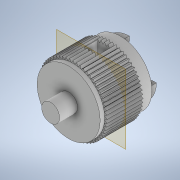
# Autodesk Inventor part: PotAttachmentB10L
Saved by Autodesk Inventor 2022 (Build 260153000, 153)
## iProperties
Created: 2021-10-23
Part Number: PotAttachmentB10L
Material: Generic
Document SubType Name: Modeling
Designer: teh18
Density: 1 g/cm^3
Appearance: Default
Author: teh18
Autodesk Inventor part; units mm, degrees
ref_plane "YZ Plane" through (0, 0, 0) normal (1, 0, 0) x (0, 1, 0)
ref_plane "XZ Plane" through (0, 0, 0) normal (0, 1, 0) x (-1, 0, 0)
ref_plane "XY Plane" through (0, 0, 0) normal (0, 0, 1) x (1, 0, 0)
sketch "Sketch1" plane through (0, 0, 0) normal (0, 0, 1) x (1, 0, 0)
  arc A0 (-0.1225, 6.9989) -> (-6, 3.6056) centre (0, 0) ccw projected
  circle A1 centre (0, 0) radius 7
  line L0 (0, -12) -> (0, -10) projected
  arc A2 (0, -10) -> (10, 0) centre (0, 0) ccw projected
  line L1 (10, 0) -> (12, 0) projected
  arc A3 (0, -12) -> (12, 0) centre (0, 0) ccw projected
  line L2 (0, 12) -> (0, 10) projected
  arc A4 (0, 10) -> (-10, 0) centre (0, 0) ccw projected
  line L3 (-10, 0) -> (-12, 0) projected
  arc A5 (0, 12) -> (-12, 0) centre (0, 0) ccw projected
  arc A6 (4.4269, -19.95) -> (6.1412, -19.4907) centre (5.1647, -19.275) ccw projected
  arc A7 (13.8088, -15.0638) -> (6.1412, -19.4907) centre (12, -20.7846) ccw projected
  arc A8 (13.8088, -15.0638) -> (15.0638, -13.8088) centre (14.1103, -14.1103) ccw projected
  arc A9 (19.4907, -6.1412) -> (15.0638, -13.8088) centre (20.7846, -12) ccw projected
  arc A10 (19.4907, -6.1412) -> (19.95, -4.4269) centre (19.275, -5.1647) ccw projected
  arc A11 (27.8571, 4.5959) -> (19.95, -4.4269) centre (24, 0) ccw projected
  arc A12 (27.8571, 4.5959) -> (29.4828, 5.5468) centre (28.5, 5.3619) ccw projected
  arc A13 (29.4828, 5.5468) -> (27.5804, 11.8035) centre (0, 0) ccw projected
  line L4 (27.5804, 11.8035) -> (33.0964, 14.1643) projected
  arc A14 (33.0964, 14.1643) -> (26.445, 24.4267) centre (0, 0) ccw projected
  line L5 (26.445, 24.4267) -> (22.0375, 20.3556) projected
  arc A15 (22.0375, 20.3556) -> (-20.3556, 22.0375) centre (0, 0) ccw projected
  line L6 (-20.3556, 22.0375) -> (-16.2845, 17.63) projected
  arc A16 (-16.2845, 17.63) -> (-5.9529, -23.25) centre (0, 0) ccw projected
  arc A17 (4.4269, -19.95) -> (-5.9529, -23.25) centre (0, -24) ccw projected
  arc A18 (-1, 6.9282) -> (-6.9282, 1) centre (0, 0) ccw projected
  line L7 (-1, 6.9282) -> (-1, 1) projected
  line L8 (-1, 1) -> (-6.9282, 1) projected
  line L9 (-6.9282, -1) -> (-1, -1) projected
  line L10 (-1, -1) -> (-1, -6.9282) projected
  arc A19 (-6.9282, -1) -> (-1, -6.9282) centre (0, 0) ccw projected
  line L11 (1, -6.9282) -> (1, -1) projected
  line L12 (1, -1) -> (6.9282, -1) projected
  arc A20 (1, -6.9282) -> (6.9282, -1) centre (0, 0) ccw projected
  line L13 (6.9282, 1) -> (1, 1) projected
  line L14 (1, 1) -> (1, 6.9282) projected
  arc A21 (6.9282, 1) -> (1, 6.9282) centre (0, 0) ccw projected
  circle A22 centre (0, 0) radius 14
  point P0 (0, 0)
  point P1 (-6, 3.6056)
  point P2 (-0.1225, 6.9989)
  dimension "d2" = 28
  constraints: 1 centre point, 1 coincident, 2 other
  measures "d2" diameter of A22
extrude "Extrusion1" add sketch "Sketch1" along normal blind 23 contours L0 A2 L1 A3 | L2 A4 L3 A5 | A22
sketch "Sketch2" plane through (0, 0, 0) normal (0, 0, -1) x (-1, 0, 0)
  line L0 (0, -12) -> (0, -10) projected
  arc A0 (-10, 0) -> (0, -10) centre (0, 0) ccw projected
  line L1 (-10, 0) -> (-12, 0) projected
  arc A1 (-12, 0) -> (0, -12) centre (0, 0) ccw projected
  line L2 (0, 12) -> (0, 10) projected
  arc A2 (10, 0) -> (0, 10) centre (0, 0) ccw projected
  line L3 (10, 0) -> (12, 0) projected
  arc A3 (12, 0) -> (0, 12) centre (0, 0) ccw projected
  arc A4 (-6.1412, -19.4907) -> (-4.4269, -19.95) centre (-5.1647, -19.275) ccw projected
  arc A5 (-6.1412, -19.4907) -> (-13.8088, -15.0638) centre (-12, -20.7846) ccw projected
  arc A6 (-15.0638, -13.8088) -> (-13.8088, -15.0638) centre (-14.1103, -14.1103) ccw projected
  arc A7 (-15.0638, -13.8088) -> (-19.4907, -6.1412) centre (-20.7846, -12) ccw projected
  arc A8 (-19.95, -4.4269) -> (-19.4907, -6.1412) centre (-19.275, -5.1647) ccw projected
  arc A9 (-19.95, -4.4269) -> (-27.8571, 4.5959) centre (-24, 0) ccw projected
  arc A10 (-29.4828, 5.5468) -> (-27.8571, 4.5959) centre (-28.5, 5.3619) ccw projected
  arc A11 (-27.5804, 11.8035) -> (-29.4828, 5.5468) centre (0, 0) ccw projected
  line L4 (-27.5804, 11.8035) -> (-33.0964, 14.1643) projected
  arc A12 (-26.445, 24.4267) -> (-33.0964, 14.1643) centre (0, 0) ccw projected
  line L5 (-26.445, 24.4267) -> (-22.0375, 20.3556) projected
  arc A13 (20.3556, 22.0375) -> (-22.0375, 20.3556) centre (0, 0) ccw projected
  line L6 (20.3556, 22.0375) -> (16.2845, 17.63) projected
  arc A14 (5.9529, -23.25) -> (16.2845, 17.63) centre (0, 0) ccw projected
  arc A15 (5.9529, -23.25) -> (-4.4269, -19.95) centre (0, -24) ccw projected
  arc A16 (6.9282, 1) -> (1, 6.9282) centre (0, 0) ccw projected
  line L7 (1, 6.9282) -> (1, 1) projected
  line L8 (1, 1) -> (6.9282, 1) projected
  line L9 (6.9282, -1) -> (1, -1) projected
  line L10 (1, -1) -> (1, -6.9282) projected
  arc A17 (1, -6.9282) -> (6.9282, -1) centre (0, 0) ccw projected
  line L11 (-1, -6.9282) -> (-1, -1) projected
  line L12 (-1, -1) -> (-6.9282, -1) projected
  arc A18 (-6.9282, -1) -> (-1, -6.9282) centre (0, 0) ccw projected
  line L13 (-6.9282, 1) -> (-1, 1) projected
  line L14 (-1, 1) -> (-1, 6.9282) projected
  arc A19 (-1, 6.9282) -> (-6.9282, 1) centre (0, 0) ccw projected
  point P0 (0, 0)
extrude "Extrusion2" add sketch "Sketch2" along normal blind 4 contours A1 L1 A0 L0 | A3 L3 A2 L2
ref_plane "Work Plane1" through (0, 0, 13) normal (0, 0, 1) x (1, 0, 0)
sketch "Sketch4" plane through (0, 0, 13) normal (0, 0, 1) x (1, 0, 0)
  circle A0 centre (0, 0) radius 3
  circle A1 centre (0, 0) radius 7 projected
  dimension "d10" = 6
  constraints: 1 centre point, 1 coincident
  measures "d10" diameter of A0
extrude "Extrusion4" add sketch "Sketch4" along normal up to surface (10 mm away) contours A0 | A1
sketch "Sketch6" plane through (0, 0, 23) normal (0, 0, 1) x (1, 0, 0)
  circle A0 centre (0, 0) radius 4
  dimension "d25" = 8
  constraints: 1 centre point, 1 coincident
  measures "d25" diameter of A0
extrude "Extrusion6" add sketch "Sketch6" along normal blind 8
sketch "Sketch7" plane through (0, 0, 13) normal (0, 0, 1) x (1, 0, 0)
  circle A0 centre (0, 0) radius 14 projected
  line L0 (0, 15.1547) -> (1, 13.4226)
  line L1 (1, 13.4226) -> (-1, 13.4226)
  line L2 (-1, 13.4226) -> (0, 15.1547)
  line L3 (-1.5841, 15.0717) -> (-0.4085, 13.4536)
  line L4 (-2.3976, 13.2446) -> (-1.5841, 15.0717)
  line L5 (-0.4085, 13.4536) -> (-2.3976, 13.2446)
  line L6 (-3.1508, 14.8235) -> (-1.8126, 13.3372)
  line L7 (-3.7689, 12.9214) -> (-3.1508, 14.8235)
  line L8 (-1.8126, 13.3372) -> (-3.7689, 12.9214)
  line L9 (-4.6831, 14.413) -> (-3.1968, 13.0747)
  line L10 (-5.0989, 12.4567) -> (-4.6831, 14.413)
  line L11 (-3.1968, 13.0747) -> (-5.0989, 12.4567)
  line L12 (-6.164, 13.8445) -> (-4.5459, 12.6689)
  line L13 (-6.373, 11.8555) -> (-6.164, 13.8445)
  line L14 (-4.5459, 12.6689) -> (-6.373, 11.8555)
  line L15 (-7.5774, 13.1244) -> (-5.8453, 12.1244)
  line L16 (-7.5774, 11.1244) -> (-7.5774, 13.1244)
  line L17 (-5.8453, 12.1244) -> (-7.5774, 11.1244)
  line L18 (-8.9077, 12.2604) -> (-7.0806, 11.4469)
  line L19 (-8.6987, 10.2714) -> (-8.9077, 12.2604)
  line L20 (-7.0806, 11.4469) -> (-8.6987, 10.2714)
  line L21 (-10.1405, 11.2621) -> (-8.2384, 10.6441)
  line L22 (-9.7247, 9.3058) -> (-10.1405, 11.2621)
  line L23 (-8.2384, 10.6441) -> (-9.7247, 9.3058)
  line L24 (-11.2621, 10.1405) -> (-9.3058, 9.7247)
  line L25 (-10.6441, 8.2384) -> (-11.2621, 10.1405)
  line L26 (-9.3058, 9.7247) -> (-10.6441, 8.2384)
  line L27 (-12.2604, 8.9077) -> (-10.2714, 8.6987)
  line L28 (-11.4469, 7.0806) -> (-12.2604, 8.9077)
  line L29 (-10.2714, 8.6987) -> (-11.4469, 7.0806)
  line L30 (-13.1244, 7.5774) -> (-11.1244, 7.5774)
  line L31 (-12.1244, 5.8453) -> (-13.1244, 7.5774)
  line L32 (-11.1244, 7.5774) -> (-12.1244, 5.8453)
  line L33 (-13.8445, 6.164) -> (-11.8555, 6.373)
  line L34 (-12.6689, 4.5459) -> (-13.8445, 6.164)
  line L35 (-11.8555, 6.373) -> (-12.6689, 4.5459)
  line L36 (-14.413, 4.6831) -> (-12.4567, 5.0989)
  line L37 (-13.0747, 3.1968) -> (-14.413, 4.6831)
  line L38 (-12.4567, 5.0989) -> (-13.0747, 3.1968)
  line L39 (-14.8235, 3.1508) -> (-12.9214, 3.7689)
  line L40 (-13.3372, 1.8126) -> (-14.8235, 3.1508)
  line L41 (-12.9214, 3.7689) -> (-13.3372, 1.8126)
  line L42 (-15.0717, 1.5841) -> (-13.2446, 2.3976)
  line L43 (-13.4536, 0.4085) -> (-15.0717, 1.5841)
  line L44 (-13.2446, 2.3976) -> (-13.4536, 0.4085)
  line L45 (-15.1547, 0) -> (-13.4226, 1)
  line L46 (-13.4226, -1) -> (-15.1547, 0)
  line L47 (-13.4226, 1) -> (-13.4226, -1)
  line L48 (-15.0717, -1.5841) -> (-13.4536, -0.4085)
  line L49 (-13.2446, -2.3976) -> (-15.0717, -1.5841)
  line L50 (-13.4536, -0.4085) -> (-13.2446, -2.3976)
  line L51 (-14.8235, -3.1508) -> (-13.3372, -1.8126)
  line L52 (-12.9214, -3.7689) -> (-14.8235, -3.1508)
  line L53 (-13.3372, -1.8126) -> (-12.9214, -3.7689)
  line L54 (-14.413, -4.6831) -> (-13.0747, -3.1968)
  line L55 (-12.4567, -5.0989) -> (-14.413, -4.6831)
  line L56 (-13.0747, -3.1968) -> (-12.4567, -5.0989)
  line L57 (-13.8445, -6.164) -> (-12.6689, -4.5459)
  line L58 (-11.8555, -6.373) -> (-13.8445, -6.164)
  line L59 (-12.6689, -4.5459) -> (-11.8555, -6.373)
  line L60 (-13.1244, -7.5774) -> (-12.1244, -5.8453)
  line L61 (-11.1244, -7.5774) -> (-13.1244, -7.5774)
  line L62 (-12.1244, -5.8453) -> (-11.1244, -7.5774)
  line L63 (-12.2604, -8.9077) -> (-11.4469, -7.0806)
  line L64 (-10.2714, -8.6987) -> (-12.2604, -8.9077)
  line L65 (-11.4469, -7.0806) -> (-10.2714, -8.6987)
  line L66 (-11.2621, -10.1405) -> (-10.6441, -8.2384)
  line L67 (-9.3058, -9.7247) -> (-11.2621, -10.1405)
  line L68 (-10.6441, -8.2384) -> (-9.3058, -9.7247)
  line L69 (-10.1405, -11.2621) -> (-9.7247, -9.3058)
  line L70 (-8.2384, -10.6441) -> (-10.1405, -11.2621)
  line L71 (-9.7247, -9.3058) -> (-8.2384, -10.6441)
  line L72 (-8.9077, -12.2604) -> (-8.6987, -10.2714)
  line L73 (-7.0806, -11.4469) -> (-8.9077, -12.2604)
  line L74 (-8.6987, -10.2714) -> (-7.0806, -11.4469)
  line L75 (-7.5774, -13.1244) -> (-7.5774, -11.1244)
  line L76 (-5.8453, -12.1244) -> (-7.5774, -13.1244)
  line L77 (-7.5774, -11.1244) -> (-5.8453, -12.1244)
  line L78 (-6.164, -13.8445) -> (-6.373, -11.8555)
  line L79 (-4.5459, -12.6689) -> (-6.164, -13.8445)
  line L80 (-6.373, -11.8555) -> (-4.5459, -12.6689)
  line L81 (-4.6831, -14.413) -> (-5.0989, -12.4567)
  line L82 (-3.1968, -13.0747) -> (-4.6831, -14.413)
  line L83 (-5.0989, -12.4567) -> (-3.1968, -13.0747)
  line L84 (-3.1508, -14.8235) -> (-3.7689, -12.9214)
  line L85 (-1.8126, -13.3372) -> (-3.1508, -14.8235)
  line L86 (-3.7689, -12.9214) -> (-1.8126, -13.3372)
  line L87 (-1.5841, -15.0717) -> (-2.3976, -13.2446)
  line L88 (-0.4085, -13.4536) -> (-1.5841, -15.0717)
  line L89 (-2.3976, -13.2446) -> (-0.4085, -13.4536)
  line L90 (0, -15.1547) -> (-1, -13.4226)
  line L91 (1, -13.4226) -> (0, -15.1547)
  line L92 (-1, -13.4226) -> (1, -13.4226)
  line L93 (1.5841, -15.0717) -> (0.4085, -13.4536)
  line L94 (2.3976, -13.2446) -> (1.5841, -15.0717)
  line L95 (0.4085, -13.4536) -> (2.3976, -13.2446)
  line L96 (3.1508, -14.8235) -> (1.8126, -13.3372)
  line L97 (3.7689, -12.9214) -> (3.1508, -14.8235)
  line L98 (1.8126, -13.3372) -> (3.7689, -12.9214)
  line L99 (4.6831, -14.413) -> (3.1968, -13.0747)
  line L100 (5.0989, -12.4567) -> (4.6831, -14.413)
  line L101 (3.1968, -13.0747) -> (5.0989, -12.4567)
  line L102 (6.164, -13.8445) -> (4.5459, -12.6689)
  line L103 (6.373, -11.8555) -> (6.164, -13.8445)
  line L104 (4.5459, -12.6689) -> (6.373, -11.8555)
  line L105 (7.5774, -13.1244) -> (5.8453, -12.1244)
  line L106 (7.5774, -11.1244) -> (7.5774, -13.1244)
  line L107 (5.8453, -12.1244) -> (7.5774, -11.1244)
  line L108 (8.9077, -12.2604) -> (7.0806, -11.4469)
  line L109 (8.6987, -10.2714) -> (8.9077, -12.2604)
  line L110 (7.0806, -11.4469) -> (8.6987, -10.2714)
  line L111 (10.1405, -11.2621) -> (8.2384, -10.6441)
  line L112 (9.7247, -9.3058) -> (10.1405, -11.2621)
  line L113 (8.2384, -10.6441) -> (9.7247, -9.3058)
  line L114 (11.2621, -10.1405) -> (9.3058, -9.7247)
  line L115 (10.6441, -8.2384) -> (11.2621, -10.1405)
  line L116 (9.3058, -9.7247) -> (10.6441, -8.2384)
  line L117 (12.2604, -8.9077) -> (10.2714, -8.6987)
  line L118 (11.4469, -7.0806) -> (12.2604, -8.9077)
  line L119 (10.2714, -8.6987) -> (11.4469, -7.0806)
  line L120 (13.1244, -7.5774) -> (11.1244, -7.5774)
  line L121 (12.1244, -5.8453) -> (13.1244, -7.5774)
  line L122 (11.1244, -7.5774) -> (12.1244, -5.8453)
  line L123 (13.8445, -6.164) -> (11.8555, -6.373)
  line L124 (12.6689, -4.5459) -> (13.8445, -6.164)
  line L125 (11.8555, -6.373) -> (12.6689, -4.5459)
  line L126 (14.413, -4.6831) -> (12.4567, -5.0989)
  line L127 (13.0747, -3.1968) -> (14.413, -4.6831)
  line L128 (12.4567, -5.0989) -> (13.0747, -3.1968)
  line L129 (14.8235, -3.1508) -> (12.9214, -3.7689)
  line L130 (13.3372, -1.8126) -> (14.8235, -3.1508)
  line L131 (12.9214, -3.7689) -> (13.3372, -1.8126)
  line L132 (15.0717, -1.5841) -> (13.2446, -2.3976)
  line L133 (13.4536, -0.4085) -> (15.0717, -1.5841)
  line L134 (13.2446, -2.3976) -> (13.4536, -0.4085)
  line L135 (15.1547, 0) -> (13.4226, -1)
  line L136 (13.4226, 1) -> (15.1547, 0)
  line L137 (13.4226, -1) -> (13.4226, 1)
  line L138 (15.0717, 1.5841) -> (13.4536, 0.4085)
  line L139 (13.2446, 2.3976) -> (15.0717, 1.5841)
  line L140 (13.4536, 0.4085) -> (13.2446, 2.3976)
  line L141 (14.8235, 3.1508) -> (13.3372, 1.8126)
  line L142 (12.9214, 3.7689) -> (14.8235, 3.1508)
  line L143 (13.3372, 1.8126) -> (12.9214, 3.7689)
  line L144 (14.413, 4.6831) -> (13.0747, 3.1968)
  line L145 (12.4567, 5.0989) -> (14.413, 4.6831)
  line L146 (13.0747, 3.1968) -> (12.4567, 5.0989)
  line L147 (13.8445, 6.164) -> (12.6689, 4.5459)
  line L148 (11.8555, 6.373) -> (13.8445, 6.164)
  line L149 (12.6689, 4.5459) -> (11.8555, 6.373)
  line L150 (13.1244, 7.5774) -> (12.1244, 5.8453)
  line L151 (11.1244, 7.5774) -> (13.1244, 7.5774)
  line L152 (12.1244, 5.8453) -> (11.1244, 7.5774)
  line L153 (12.2604, 8.9077) -> (11.4469, 7.0806)
  line L154 (10.2714, 8.6987) -> (12.2604, 8.9077)
  line L155 (11.4469, 7.0806) -> (10.2714, 8.6987)
  line L156 (11.2621, 10.1405) -> (10.6441, 8.2384)
  line L157 (9.3058, 9.7247) -> (11.2621, 10.1405)
  line L158 (10.6441, 8.2384) -> (9.3058, 9.7247)
  line L159 (10.1405, 11.2621) -> (9.7247, 9.3058)
  line L160 (8.2384, 10.6441) -> (10.1405, 11.2621)
  line L161 (9.7247, 9.3058) -> (8.2384, 10.6441)
  line L162 (8.9077, 12.2604) -> (8.6987, 10.2714)
  line L163 (7.0806, 11.4469) -> (8.9077, 12.2604)
  line L164 (8.6987, 10.2714) -> (7.0806, 11.4469)
  line L165 (7.5774, 13.1244) -> (7.5774, 11.1244)
  line L166 (5.8453, 12.1244) -> (7.5774, 13.1244)
  line L167 (7.5774, 11.1244) -> (5.8453, 12.1244)
  line L168 (6.164, 13.8445) -> (6.373, 11.8555)
  line L169 (4.5459, 12.6689) -> (6.164, 13.8445)
  line L170 (6.373, 11.8555) -> (4.5459, 12.6689)
  line L171 (4.6831, 14.413) -> (5.0989, 12.4567)
  line L172 (3.1968, 13.0747) -> (4.6831, 14.413)
  line L173 (5.0989, 12.4567) -> (3.1968, 13.0747)
  line L174 (3.1508, 14.8235) -> (3.7689, 12.9214)
  line L175 (1.8126, 13.3372) -> (3.1508, 14.8235)
  line L176 (3.7689, 12.9214) -> (1.8126, 13.3372)
  line L177 (1.5841, 15.0717) -> (2.3976, 13.2446)
  line L178 (0.4085, 13.4536) -> (1.5841, 15.0717)
  line L179 (2.3976, 13.2446) -> (0.4085, 13.4536)
  point P0 (0, 0)
  point P1 (0, 14)
  point P2 (-1.4634, 13.9233)
  point P3 (-2.9108, 13.6941)
  point P4 (-4.3262, 13.3148)
  point P5 (-5.6943, 12.7896)
  point P6 (-7, 12.1244)
  point P7 (-8.229, 11.3262)
  point P8 (-9.3678, 10.404)
  point P9 (-10.404, 9.3678)
  point P10 (-11.3262, 8.229)
  point P11 (-12.1244, 7)
  point P12 (-12.7896, 5.6943)
  point P13 (-13.3148, 4.3262)
  point P14 (-13.6941, 2.9108)
  point P15 (-13.9233, 1.4634)
  point P16 (-14, 0)
  point P17 (-13.9233, -1.4634)
  point P18 (-13.6941, -2.9108)
  point P19 (-13.3148, -4.3262)
  point P20 (-12.7896, -5.6943)
  point P21 (-12.1244, -7)
  point P22 (-11.3262, -8.229)
  point P23 (-10.404, -9.3678)
  point P24 (-9.3678, -10.404)
  point P25 (-8.229, -11.3262)
  point P26 (-7, -12.1244)
  point P27 (-5.6943, -12.7896)
  point P28 (-4.3262, -13.3148)
  point P29 (-2.9108, -13.6941)
  point P30 (-1.4634, -13.9233)
  point P31 (0, -14)
  point P32 (1.4634, -13.9233)
  point P33 (2.9108, -13.6941)
  point P34 (4.3262, -13.3148)
  point P35 (5.6943, -12.7896)
  point P36 (7, -12.1244)
  point P37 (8.229, -11.3262)
  point P38 (9.3678, -10.404)
  point P39 (10.404, -9.3678)
  point P40 (11.3262, -8.229)
  point P41 (12.1244, -7)
  point P42 (12.7896, -5.6943)
  point P43 (13.3148, -4.3262)
  point P44 (13.6941, -2.9108)
  point P45 (13.9233, -1.4634)
  point P46 (14, 0)
  point P47 (13.9233, 1.4634)
  point P48 (13.6941, 2.9108)
  point P49 (13.3148, 4.3262)
  point P50 (12.7896, 5.6943)
  point P51 (12.1244, 7)
  point P52 (11.3262, 8.229)
  point P53 (10.404, 9.3678)
  point P54 (9.3678, 10.404)
  point P55 (8.229, 11.3262)
  point P56 (7, 12.1244)
  point P57 (5.6943, 12.7896)
  point P58 (4.3262, 13.3148)
  point P59 (2.9108, 13.6941)
  point P60 (1.4634, 13.9233)
  point P61 (2.246, 13.8187)
  point P62 (2.1341, 13.8364)
  point P63 (0.7893, 13.9777)
  point P64 (0.6761, 13.9837)
  point P65 (-0.6761, 13.9837)
  point P66 (-0.7893, 13.9777)
  point P67 (-2.1341, 13.8364)
  point P68 (-2.246, 13.8187)
  point P69 (-3.5687, 13.5375)
  point P70 (-3.6782, 13.5082)
  point P71 (-4.9642, 13.0903)
  point P72 (-5.07, 13.0497)
  point P73 (-6.3053, 12.4997)
  point P74 (-6.4063, 12.4483)
  point P75 (-7.5774, 11.7722)
  point P76 (-7.6724, 11.7104)
  point P77 (-8.7664, 10.9156)
  point P78 (-8.8545, 10.8443)
  point P79 (-9.8593, 9.9395)
  point P80 (-9.9395, 9.8593)
  point P81 (-10.8443, 8.8545)
  point P82 (-10.9156, 8.7664)
  point P83 (-11.7104, 7.6724)
  point P84 (-11.7722, 7.5774)
  point P85 (-12.4483, 6.4063)
  point P86 (-12.4997, 6.3053)
  point P87 (-13.0497, 5.07)
  point P88 (-13.0903, 4.9642)
  point P89 (-13.5082, 3.6782)
  point P90 (-13.5375, 3.5687)
  point P91 (-13.8187, 2.246)
  point P92 (-13.8364, 2.1341)
  point P93 (-13.9777, 0.7893)
  point P94 (-13.9837, 0.6761)
  point P95 (-13.9837, -0.6761)
  point P96 (-13.9777, -0.7893)
  point P97 (-13.8364, -2.1341)
  point P98 (-13.8187, -2.246)
  point P99 (-13.5375, -3.5687)
  point P100 (-13.5082, -3.6782)
  point P101 (-13.0903, -4.9642)
  point P102 (-13.0497, -5.07)
  point P103 (-12.4997, -6.3053)
  point P104 (-12.4483, -6.4063)
  point P105 (-11.7722, -7.5774)
  point P106 (-11.7104, -7.6724)
  point P107 (-10.9156, -8.7664)
  point P108 (-10.8443, -8.8545)
  point P109 (-9.9395, -9.8593)
  point P110 (-9.8593, -9.9395)
  point P111 (-8.8545, -10.8443)
  point P112 (-8.7664, -10.9156)
  point P113 (-7.6724, -11.7104)
  point P114 (-7.5774, -11.7722)
  point P115 (-6.4063, -12.4483)
  point P116 (-6.3053, -12.4997)
  point P117 (-5.07, -13.0497)
  point P118 (-4.9642, -13.0903)
  point P119 (-3.6782, -13.5082)
  point P120 (-3.5687, -13.5375)
  point P121 (-2.246, -13.8187)
  point P122 (-2.1341, -13.8364)
  point P123 (-0.7893, -13.9777)
  point P124 (-0.6761, -13.9837)
  point P125 (0.6761, -13.9837)
  point P126 (0.7893, -13.9777)
  point P127 (2.1341, -13.8364)
  point P128 (2.246, -13.8187)
  point P129 (3.5687, -13.5375)
  point P130 (3.6782, -13.5082)
  point P131 (4.9642, -13.0903)
  point P132 (5.07, -13.0497)
  point P133 (6.3053, -12.4997)
  point P134 (6.4063, -12.4483)
  point P135 (7.5774, -11.7722)
  point P136 (7.6724, -11.7104)
  point P137 (8.7664, -10.9156)
  point P138 (8.8545, -10.8443)
  point P139 (9.8593, -9.9395)
  point P140 (9.9395, -9.8593)
  point P141 (10.8443, -8.8545)
  point P142 (10.9156, -8.7664)
  point P143 (11.7104, -7.6724)
  point P144 (11.7722, -7.5774)
  point P145 (12.4483, -6.4063)
  point P146 (12.4997, -6.3053)
  point P147 (13.0497, -5.07)
  point P148 (13.0903, -4.9642)
  point P149 (13.5082, -3.6782)
  point P150 (13.5375, -3.5687)
  point P151 (13.8187, -2.246)
  point P152 (13.8364, -2.1341)
  point P153 (13.9777, -0.7893)
  point P154 (13.9837, -0.6761)
  point P155 (13.9837, 0.6761)
  point P156 (13.9777, 0.7893)
  point P157 (13.8364, 2.1341)
  point P158 (13.8187, 2.246)
  point P159 (13.5375, 3.5687)
  point P160 (13.5082, 3.6782)
  point P161 (13.0903, 4.9642)
  point P162 (13.0497, 5.07)
  point P163 (12.4997, 6.3053)
  point P164 (12.4483, 6.4063)
  point P165 (11.7722, 7.5774)
  point P166 (11.7104, 7.6724)
  point P167 (10.9156, 8.7664)
  point P168 (10.8443, 8.8545)
  point P169 (9.9395, 9.8593)
  point P170 (9.8593, 9.9395)
  point P171 (8.8545, 10.8443)
  point P172 (8.7664, 10.9156)
  point P173 (7.6724, 11.7104)
  point P174 (7.5774, 11.7722)
  point P175 (6.4063, 12.4483)
  point P176 (6.3053, 12.4997)
  point P177 (5.07, 13.0497)
  point P178 (4.9642, 13.0903)
  point P179 (3.6782, 13.5082)
  point P180 (3.5687, 13.5375)
  point P181 (-0.7035, 13.4226)
  point P182 (0.7035, 13.4226)
  point P183 (2.1026, 13.2756)
  point P184 (3.4788, 12.9831)
  point P185 (4.8168, 12.5483)
  point P186 (6.1021, 11.9761)
  point P187 (7.3205, 11.2726)
  point P188 (8.4587, 10.4457)
  point P189 (9.5043, 9.5043)
  point P190 (10.4457, 8.4587)
  point P191 (11.2726, 7.3205)
  point P192 (11.9761, 6.1021)
  point P193 (12.5483, 4.8168)
  point P194 (12.9831, 3.4788)
  point P195 (13.2756, 2.1026)
  point P196 (13.4226, 0.7035)
  point P197 (13.4226, -0.7035)
  point P198 (13.2756, -2.1026)
  point P199 (12.9831, -3.4788)
  dimension "d28" = 2
  dimension "d31" = 360
  constraints: 360 end point, 1 horizontal alignment, 1 vertical alignment, 429 other
  measures "d28" distance of L0.end L1.end
extrude "Extrusion7" add sketch "Sketch7" along normal mid plane 16 contours A0 L135 L133 L134 L137 L140 L138 L136 | A0 L136 L135 | L136 L138 A0 | A0 L133 L135 | L138 L136 L137 L140 L143 L141 L139 A0 | A0 L139 L138 | L138 L140 L137 L136 | L133 L132 A0 | A0 L132 L130 L131 L134 L137 L135 L133 | L135 L137 L134 L133 | L139 L141 A0 | A0 L130 L132 | L141 L139 L140 L143 L146 L144 L142 A0 | A0 L142 L141 | L141 L143 L140 L139 | L130 L129 A0 | A0 L129 L127 L128 L131 L134 L132 L130 | L132 L134 L131 L130 | L142 L144 A0 | A0 L127 L129 | L144 L142 L143 L146 L149 L147 L145 A0 | A0 L145 L144 | L144 L146 L143 L142 | L127 L126 A0 | A0 L126 L124 L125 L128 L131 L129 L127 | L129 L131 L128 L127 | L145 L147 A0 | L149 L152 L150 L148 A0 L147 L145 L146 | L146 L145 L147 L149 | A0 L124 L126 | L128 L126 L124 A0 L123 L121 L122 L125 | L125 L124 L126 L128 | A0 L148 L147 | L152 L155 L153 L151 A0 L150 L148 L149 | L149 L148 L150 L152 | L124 L123 A0 | L125 L123 L121 A0 L120 L118 L119 L122 | L122 L121 L123 L125 | L148 L150 A0 | L155 L158 L156 L154 A0 L153 L151 L152 | L152 L151 L153 L155 | A0 L121 L123 | L122 L120 L118 A0 L117 L115 L116 L119 | L119 L118 L120 L122 | A0 L151 L150 | L158 L161 L159 L157 A0 L156 L154 L155 | L155 L154 L156 L158 | L121 L120 A0 | L119 L117 L115 A0 L114 L112 L113 L116 | L116 L115 L117 L119 | L151 L153 A0 | L161 L164 L162 L160 A0 L159 L157 L158 | L158 L157 L159 L161 | A0 L118 L120 | L116 L114 L112 A0 L111 L109 L110 L113 | L113 L112 L114 L116 | A0 L154 L153 | L156 A0 L154 | L164 L167 L165 L163 A0 L162 L160 L161 | L161 L160 L162 L164 | L118 L117 A0 | L113 L111 L109 A0 L108 L106 L107 L110 | L110 L109 L111 L113 | L117 A0 L115 | A0 L157 L156 | L159 A0 L157 | L167 L170 L168 L166 A0 L165 L163 L164 | L164 L163 L165 L167 | L110 L108 L106 A0 L105 L103 L104 L107 | L107 L106 L108 L110 | L114 A0 L112 | L115 L114 A0 | A0 L160 L159 | L162 A0 L160 | L170 L173 L171 L169 A0 L168 L166 L167 | L167 L166 L168 L170 | L107 L105 L103 A0 L102 L100 L101 L104 | L104 L103 L105 L107 | L111 A0 L109 | L112 L111 A0 | A0 L163 L162 | L165 A0 L163 | L173 L176 L174 L172 A0 L171 L169 L170 | L170 L169 L171 L173 | L104 L102 L100 A0 L99 L97 L98 L101 | L101 L100 L102 L104 | L108 A0 L106 | L109 L108 A0 | A0 L166 L165 | L168 A0 L166 | L176 L179 L177 L175 A0 L174 L172 L173 | L173 L172 L174 L176 | L101 L99 L97 A0 L96 L94 L95 L98 | L98 L97 L99 L101 | L105 A0 L103 | L106 L105 A0 | A0 L169 L168 | L171 A0 L169 | L179 L1 L0 L178 A0 L177 L175 L176 | L176 L175 L177 L179 | L98 L96 L94 A0 L93 L91 L92 L95 | L95 L94 L96 L98 | L102 A0 L100 | L103 L102 A0 | A0 L172 L171 | L174 A0 L172 | L179 L178 L0 L1 | L1 L5 L3 L2 A0 L0 L178 L179 | L95 L93 L91 A0 L90 L88 L89 L92 | L92 L91 L93 L95 | L99 A0 L97 | L100 L99 A0 | A0 L175 L174 | L177 A0 L175 | L5 L8 L6 L4 A0 L3 L2 L1 | L1 L2 L3 L5 | L92 L90 L88 A0 L87 L85 L86 L89 | L89 L88 L90 L92 | L96 A0 L94 | L97 L96 A0 | A0 L178 L177 | L0 A0 L178 | L8 L11 L9 L7 A0 L6 L4 L5 | L5 L4 L6 L8 | L89 L87 L85 A0 L84 L82 L83 L86 | L86 L85 L87 L89 | L93 A0 L91 | L94 L93 A0 | A0 L2 L0 | L3 A0 L2 | L11 L14 L12 L10 A0 L9 L7 L8 | L8 L7 L9 L11 | L86 L84 L82 A0 L81 L79 L80 L83 | L83 L82 L84 L86 | L90 A0 L88 | L91 L90 A0 | A0 L4 L3 | L6 A0 L4 | L14 L17 L15 L13 A0 L12 L10 L11 | L11 L10 L12 L14 | L83 L81 L79 A0 L78 L76 L77 L80 | L80 L79 L81 L83 | L87 A0 L85 | L88 L87 A0 | A0 L7 L6 | L9 A0 L7 | L17 L20 L18 L16 A0 L15 L13 L14 | L14 L13 L15 L17 | L80 L78 L76 A0 L75 L73 L74 L77 | L77 L76 L78 L80 | L84 A0 L82 | L85 L84 A0 | A0 L10 L9 | L12 A0 L10 | L20 L23 L21 L19 A0 L18 L16 L17 | L17 L16 L18 L20 | L77 L75 L73 A0 L72 L70 L71 L74 | L74 L73 L75 L77 | L81 A0 L79 | L82 L81 A0 | A0 L13 L12 | L15 A0 L13 | L23 L26 L24 L22 A0 L21 L19 L20 | L20 L19 L21 L23 | L74 L72 L70 A0 L69 L67 L68 L71 | L71 L70 L72 L74 | L78 A0 L76 | L79 L78 A0 | A0 L16 L15 | L18 A0 L16 | L26 L29 L27 L25 A0 L24 L22 L23 | L23 L22 L24 L26 | L71 L69 L67 A0 L66 L64 L65 L68 | L68 L67 L69 L71 | L75 A0 L73 | L76 L75 A0 | A0 L19 L18 | L21 A0 L19 | L29 L32 L30 L28 A0 L27 L25 L26 | L26 L25 L27 L29 | L68 L66 L64 A0 L63 L61 L62 L65 | L65 L64 L66 L68 | L72 A0 L70 | L73 L72 A0 | A0 L22 L21 | L24 A0 L22 | L32 L35 L33 L31 A0 L30 L28 L29 | L29 L28 L30 L32 | L65 L63 L61 A0 L60 L58 L59 L62 | L62 L61 L63 L65 | L69 A0 L67 | L70 L69 A0 | A0 L25 L24 | L27 A0 L25 | L35 L38 L36 L34 A0 L33 L31 L32 | L32 L31 L33 L35 | L62 L60 L58 A0 L57 L55 L56 L59 | L59 L58 L60 L62 | L66 A0 L64 | L67 L66 A0 | A0 L28 L27 | L30 A0 L28 | L38 L41 L39 L37 A0 L36 L34 L35 | L35 L34 L36 L38 | L59 L57 L55 A0 L54 L52 L53 L56 | L56 L55 L57 L59 | L63 A0 L61 | L64 L63 A0 | A0 L31 L30 | L33 A0 L31 | L41 L44 L42 L40 A0 L39 L37 L38 | L38 L37 L39 L41 | L56 L54 L52 A0 L51 L49 L50 L53 | L53 L52 L54 L56 | L60 A0 L58 | L61 L60 A0 | A0 L34 L33 | L36 A0 L34 | L44 L47 L45 L43 A0 L42 L40 L41 | L41 L40 L42 L44 | L53 L51 L49 A0 L48 L46 L47 L50 | L50 L49 L51 L53 | L57 A0 L55 | L58 L57 A0 | A0 L37 L36 | L39 A0 L37 | L47 L50 L48 L46 A0 L45 L43 L44 | L44 L43 L45 L47 | L47 L46 L48 L50 | L54 A0 L52 | L55 L54 A0 | A0 L40 L39 | L42 A0 L40 | L51 A0 L49 | L52 L51 A0 | A0 L43 L42 | L45 A0 L43 | L48 A0 L46 | L49 L48 A0 | A0 L46 L45
sketch "Sketch5" plane through (0, 0, 13) normal (0, 0, 1) x (1, 0, 0)
  line L0 (-3, 21.8882) -> (3, 21.8882)
  line L1 (3, 21.8882) -> (3, 3)
  line L2 (3, 3) -> (-3, 3)
  line L3 (-3, 3) -> (-3, 21.8882)
  line L4 (-3, 21.8882) -> (3, 3) construction
  line L5 (3, 21.8882) -> (-3, 3) construction
  arc A0 (3, 0) -> (3, 0) centre (0, 0) ccw projected
  point P0 (0, 12.4441)
  dimension "d14" = 6
  constraints: 12 end point, 2 midpoint, 2 parallel, 1 horizontal, 1 perpendicular
  measures "d14" distance of L1.end L2.end
extrude "Extrusion5" cut sketch "Sketch5" against normal blind 6 contours L0 L1 L2 L3
body "Solid1"
